Autodesk Inventor part; units mm, degrees
(part 2 of 2)
sketch "Skizze6" plane through (0, 0, -1.5) normal (0, 0, -1) x (-1, 0, 0)
  arc A0 (49.257, 13.1596) -> (46.9701, 10.7429) centre (49.9272, 10.235) ccw projected
  line L0 (49.257, 13.1596) -> (61.5242, 15.8801) projected
  arc A1 (63.0188, 15.8297) -> (61.5242, 15.8801) centre (62.1736, 12.9516) ccw projected
  line L1 (63.0188, 15.8297) -> (83.4642, 9.8255) projected
  arc A2 (83.4642, 9.8255) -> (85.086, 9.8061) centre (84.3096, 12.7044) ccw projected
  line L2 (85.086, 9.8061) -> (103.3977, 14.7128) projected
  arc A3 (103.3977, 14.7128) -> (105.5192, 18.3871) centre (102.6211, 17.6108) ccw projected
  line L3 (105.5192, 18.3871) -> (91.019, 72.5018) projected
  arc A4 (91.019, 72.5018) -> (88.8338, 74.6394) centre (88.1214, 71.7253) ccw projected
  line L4 (88.8338, 74.6394) -> (63.1786, 80.9125) projected
  arc A5 (63.1786, 80.9125) -> (62.6219, 80.9928) centre (62.4855, 78.0777) ccw projected
  line L5 (62.6219, 80.9928) -> (42.9227, 81.9679) projected
  arc A6 (42.9227, 81.9679) -> (41.7484, 81.7906) centre (42.7745, 78.9724) ccw projected
  line L6 (41.7484, 81.7906) -> (21.3272, 74.3579) projected
  arc A7 (21.3272, 74.3579) -> (20.5259, 73.9182) centre (22.3538, 71.5374) ccw projected
  line L7 (20.5259, 73.9182) -> (5.3305, 62.2476) projected
  arc A8 (4.8188, 61.9306) -> (5.3305, 62.2476) centre (3.5014, 64.629) ccw projected
  line L8 (4.8188, 61.9306) -> (-10.8605, 54.2803) projected
  arc A9 (-12.7723, 53.6855) -> (-10.8605, 54.2803) centre (-13.7536, 60.2096) ccw projected
  line L9 (-12.7723, 53.6855) -> (-36.149, 53.6855) projected
  arc A10 (-38.0608, 54.2803) -> (-36.149, 53.6855) centre (-36.149, 57.0556) ccw projected
  line L10 (-38.0608, 54.2803) -> (-53.7401, 61.9306) projected
  arc A11 (-54.2518, 62.2476) -> (-53.7401, 61.9306) centre (-52.4258, 64.6241) ccw projected
  line L11 (-54.2518, 62.2476) -> (-69.4472, 73.9182) projected
  arc A12 (-69.4472, 73.9182) -> (-70.2485, 74.3579) centre (-71.2736, 71.5402) ccw projected
  line L12 (-70.2485, 74.3579) -> (-90.6697, 81.7906) projected
  arc A13 (-90.6697, 81.7906) -> (-91.8441, 81.9679) centre (-91.696, 78.9707) ccw projected
  line L13 (-91.8441, 81.9679) -> (-111.5432, 80.9928) projected
  arc A14 (-111.5432, 80.9928) -> (-112.0999, 80.9125) centre (-111.3949, 77.9952) ccw projected
  line L14 (-112.0999, 80.9125) -> (-137.7551, 74.6394) projected
  arc A15 (-137.7551, 74.6394) -> (-139.9403, 72.5018) centre (-137.0425, 71.7251) ccw projected
  line L15 (-139.9403, 72.5018) -> (-154.4405, 18.3871) projected
  arc A16 (-154.4405, 18.3871) -> (-152.319, 14.7128) centre (-151.5428, 17.6106) ccw projected
  line L16 (-152.319, 14.7128) -> (-134.0073, 9.8061) projected
  arc A17 (-134.0073, 9.8061) -> (-132.3855, 9.8255) centre (-133.2309, 12.7035) ccw projected
  line L17 (-132.3855, 9.8255) -> (-111.9401, 15.8297) projected
  arc A18 (-110.4455, 15.8801) -> (-111.9401, 15.8297) centre (-111.0949, 12.9519) ccw projected
  line L18 (-110.4455, 15.8801) -> (-98.1783, 13.1596) projected
  arc A19 (-95.8914, 10.7429) -> (-98.1783, 13.1596) centre (-98.8211, 10.2609) ccw projected
  line L19 (-95.8914, 10.7429) -> (-92.4348, -9.3825) projected
  arc A20 (-92.4348, -9.3825) -> (-90.4875, -11.6997) centre (-89.4782, -8.8747) ccw projected
  line L20 (-90.4875, -11.6997) -> (-74.5563, -17.3936) projected
  arc A21 (-72.7201, -18.4315) -> (-74.5563, -17.3936) centre (-76.6396, -23.2223) ccw projected
  line L21 (-72.7201, -18.4315) -> (-58.4773, -34.2497) projected
  arc A22 (-57.7859, -35.5723) -> (-58.4773, -34.2497) centre (-60.7074, -36.2577) ccw projected
  line L22 (-57.7859, -35.5723) -> (-53.938, -51.3943) projected
  arc A23 (-53.938, -51.3943) -> (-50.2976, -53.5965) centre (-51.0229, -50.6854) ccw projected
  line L23 (-50.2976, -53.5965) -> (-31.4601, -48.8997) projected
  arc A24 (-30.7343, -48.8106) -> (-31.4601, -48.8997) centre (-30.7343, -51.8105) ccw projected
  line L24 (-30.7343, -48.8106) -> (-18.187, -48.8106) projected
  arc A25 (-17.4612, -48.8997) -> (-18.187, -48.8106) centre (-18.187, -51.8105) ccw projected
  line L25 (-17.4612, -48.8997) -> (1.3763, -53.5965) projected
  arc A26 (1.3763, -53.5965) -> (5.0167, -51.3943) centre (2.1019, -50.686) ccw projected
  line L26 (5.0167, -51.3943) -> (8.8645, -35.5723) projected
  arc A27 (9.556, -34.2497) -> (8.8645, -35.5723) centre (11.8759, -36.3046) ccw projected
  line L27 (9.556, -34.2497) -> (23.7988, -18.4315) projected
  arc A28 (25.635, -17.3936) -> (23.7988, -18.4315) centre (26.2659, -20.6529) ccw projected
  line L28 (25.635, -17.3936) -> (41.5662, -11.6997) projected
  arc A29 (41.5662, -11.6997) -> (43.5135, -9.3825) centre (40.5563, -8.8742) ccw projected
  line L29 (43.5135, -9.3825) -> (46.9701, 10.7429) projected
  line L30 (96.6013, 36.5996) -> (82.1125, 32.7172) projected
  line L31 (82.1125, 32.7172) -> (78.2301, 47.2061) projected
  line L32 (78.2301, 47.2061) -> (92.719, 51.0885) projected
  line L33 (92.719, 51.0885) -> (96.6013, 36.5996) projected
  line L34 (45.117, 62.9038) -> (31.0217, 57.7735) projected
  line L35 (31.0217, 57.7735) -> (25.8914, 71.8689) projected
  line L36 (25.8914, 71.8689) -> (39.9867, 76.9992) projected
  line L37 (39.9867, 76.9992) -> (45.117, 62.9038) projected
  line L38 (21.718, 27.7828) -> (16.5877, 41.8782) projected
  line L39 (16.5877, 41.8782) -> (30.6831, 47.0085) projected
  line L40 (30.6831, 47.0085) -> (35.8134, 32.9131) projected
  line L41 (35.8134, 32.9131) -> (21.718, 27.7828) projected
  line L42 (5.916, 15.6462) -> (20.0113, 20.7765) projected
  line L43 (20.0113, 20.7765) -> (25.1417, 6.6811) projected
  line L44 (25.1417, 6.6811) -> (11.0463, 1.5508) projected
  line L45 (11.0463, 1.5508) -> (5.916, 15.6462) projected
  line L46 (18.6433, 24.5353) -> (4.5479, 19.405) projected
  line L47 (4.5479, 19.405) -> (-0.5824, 33.5004) projected
  line L48 (-0.5824, 33.5004) -> (13.513, 38.6307) projected
  line L49 (13.513, 38.6307) -> (18.6433, 24.5353) projected
  line L50 (15.2196, 45.6369) -> (10.0893, 59.7323) projected
  line L51 (10.0893, 59.7323) -> (24.1847, 64.8626) projected
  line L52 (24.1847, 64.8626) -> (29.315, 50.7672) projected
  line L53 (29.315, 50.7672) -> (15.2196, 45.6369) projected
  line L54 (64.6087, 21.046) -> (59.4784, 35.1414) projected
  line L55 (59.4784, 35.1414) -> (73.5738, 40.2717) projected
  line L56 (73.5738, 40.2717) -> (78.7041, 26.1763) projected
  line L57 (78.7041, 26.1763) -> (64.6087, 21.046) projected
  line L58 (91.6837, 54.9522) -> (77.1948, 51.0698) projected
  line L59 (77.1948, 51.0698) -> (73.3125, 65.5587) projected
  line L60 (73.3125, 65.5587) -> (87.8013, 69.441) projected
  line L61 (87.8013, 69.441) -> (91.6837, 54.9522) projected
  line L62 (51.612, 56.7543) -> (46.4817, 70.8497) projected
  line L63 (46.4817, 70.8497) -> (60.5771, 75.98) projected
  line L64 (60.5771, 75.98) -> (65.7074, 61.8846) projected
  line L65 (65.7074, 61.8846) -> (51.612, 56.7543) projected
  line L66 (51.6154, 45.0496) -> (37.52, 39.9193) projected
  line L67 (37.52, 39.9193) -> (32.3897, 54.0147) projected
  line L68 (32.3897, 54.0147) -> (46.4851, 59.145) projected
  line L69 (46.4851, 59.145) -> (51.6154, 45.0496) projected
  line L70 (23.0861, 24.024) -> (37.1815, 29.1543) projected
  line L71 (37.1815, 29.1543) -> (42.3118, 15.0589) projected
  line L72 (42.3118, 15.0589) -> (28.2164, 9.9286) projected
  line L73 (28.2164, 9.9286) -> (23.0861, 24.024) projected
  line L74 (19.0184, 0.2419) -> (33.1433, 5.2903) projected
  line L75 (33.1433, 5.2903) -> (38.1917, -8.8346) projected
  line L76 (38.1917, -8.8346) -> (24.0668, -13.883) projected
  line L77 (24.0668, -13.883) -> (19.0184, 0.2419) projected
  line L78 (12.1449, 42.3895) -> (-1.9505, 37.2592) projected
  line L79 (-1.9505, 37.2592) -> (-7.0808, 51.3545) projected
  line L80 (-7.0808, 51.3545) -> (7.0146, 56.4848) projected
  line L81 (7.0146, 56.4848) -> (12.1449, 42.3895) projected
  line L82 (38.8881, 36.1605) -> (52.9835, 41.2908) projected
  line L83 (52.9835, 41.2908) -> (58.1138, 27.1954) projected
  line L84 (58.1138, 27.1954) -> (44.0184, 22.0651) projected
  line L85 (44.0184, 22.0651) -> (38.8881, 36.1605) projected
  line L86 (58.1104, 38.9001) -> (52.9801, 52.9955) projected
  line L87 (52.9801, 52.9955) -> (67.0754, 58.1258) projected
  line L88 (67.0754, 58.1258) -> (72.2057, 44.0304) projected
  line L89 (72.2057, 44.0304) -> (58.1104, 38.9001) projected
  line L90 (83.1478, 28.8535) -> (97.6366, 32.7359) projected
  line L91 (97.6366, 32.7359) -> (101.519, 18.247) projected
  line L92 (101.519, 18.247) -> (87.0301, 14.3647) projected
  line L93 (87.0301, 14.3647) -> (83.1478, 28.8535) projected
  line L94 (-127.1514, 47.2061) -> (-131.0338, 32.7172) projected
  line L95 (-131.0338, 32.7172) -> (-145.5226, 36.5996) projected
  line L96 (-145.5226, 36.5996) -> (-141.6403, 51.0885) projected
  line L97 (-141.6403, 51.0885) -> (-127.1514, 47.2061) projected
  line L98 (-74.8127, 71.8689) -> (-79.943, 57.7735) projected
  line L99 (-79.943, 57.7735) -> (-94.0383, 62.9038) projected
  line L100 (-94.0383, 62.9038) -> (-88.908, 76.9992) projected
  line L101 (-88.908, 76.9992) -> (-74.8127, 71.8689) projected
  line L102 (-79.6044, 47.0085) -> (-65.509, 41.8782) projected
  line L103 (-65.509, 41.8782) -> (-70.6393, 27.7828) projected
  line L104 (-70.6393, 27.7828) -> (-84.7347, 32.9131) projected
  line L105 (-84.7347, 32.9131) -> (-79.6044, 47.0085) projected
  line L106 (-74.063, 6.6811) -> (-68.9327, 20.7765) projected
  line L107 (-68.9327, 20.7765) -> (-54.8373, 15.6462) projected
  line L108 (-54.8373, 15.6462) -> (-59.9676, 1.5508) projected
  line L109 (-59.9676, 1.5508) -> (-74.063, 6.6811) projected
  line L110 (-48.3389, 33.5004) -> (-53.4692, 19.405) projected
  line L111 (-53.4692, 19.405) -> (-67.5646, 24.5353) projected
  line L112 (-67.5646, 24.5353) -> (-62.4343, 38.6307) projected
  line L113 (-62.4343, 38.6307) -> (-48.3389, 33.5004) projected
  line L114 (-73.106, 64.8626) -> (-59.0106, 59.7323) projected
  line L115 (-59.0106, 59.7323) -> (-64.1409, 45.6369) projected
  line L116 (-64.1409, 45.6369) -> (-78.2363, 50.7672) projected
  line L117 (-78.2363, 50.7672) -> (-73.106, 64.8626) projected
  line L118 (-122.4951, 40.2717) -> (-108.3997, 35.1414) projected
  line L119 (-108.3997, 35.1414) -> (-113.53, 21.046) projected
  line L120 (-113.53, 21.046) -> (-127.6254, 26.1763) projected
  line L121 (-127.6254, 26.1763) -> (-122.4951, 40.2717) projected
  line L122 (-122.2338, 65.5587) -> (-126.1161, 51.0698) projected
  line L123 (-126.1161, 51.0698) -> (-140.605, 54.9522) projected
  line L124 (-140.605, 54.9522) -> (-136.7226, 69.441) projected
  line L125 (-136.7226, 69.441) -> (-122.2338, 65.5587) projected
  line L126 (-109.4984, 75.98) -> (-95.403, 70.8497) projected
  line L127 (-95.403, 70.8497) -> (-100.5333, 56.7543) projected
  line L128 (-100.5333, 56.7543) -> (-114.6287, 61.8846) projected
  line L129 (-114.6287, 61.8846) -> (-109.4984, 75.98) projected
  line L130 (-81.311, 54.0147) -> (-86.4413, 39.9193) projected
  line L131 (-86.4413, 39.9193) -> (-100.5367, 45.0496) projected
  line L132 (-100.5367, 45.0496) -> (-95.4064, 59.145) projected
  line L133 (-95.4064, 59.145) -> (-81.311, 54.0147) projected
  line L134 (-91.2331, 15.0589) -> (-86.1028, 29.1543) projected
  line L135 (-86.1028, 29.1543) -> (-72.0074, 24.024) projected
  line L136 (-72.0074, 24.024) -> (-77.1377, 9.9286) projected
  line L137 (-77.1377, 9.9286) -> (-91.2331, 15.0589) projected
  line L138 (-87.113, -8.8346) -> (-82.0646, 5.2903) projected
  line L139 (-82.0646, 5.2903) -> (-67.9397, 0.2419) projected
  line L140 (-67.9397, 0.2419) -> (-72.9881, -13.883) projected
  line L141 (-72.9881, -13.883) -> (-87.113, -8.8346) projected
  line L142 (-41.8405, 51.3545) -> (-46.9708, 37.2592) projected
  line L143 (-46.9708, 37.2592) -> (-61.0662, 42.3895) projected
  line L144 (-61.0662, 42.3895) -> (-55.9359, 56.4848) projected
  line L145 (-55.9359, 56.4848) -> (-41.8405, 51.3545) projected
  line L146 (-107.0351, 27.1954) -> (-101.9048, 41.2908) projected
  line L147 (-101.9048, 41.2908) -> (-87.8094, 36.1605) projected
  line L148 (-87.8094, 36.1605) -> (-92.9397, 22.0651) projected
  line L149 (-92.9397, 22.0651) -> (-107.0351, 27.1954) projected
  line L150 (-115.9967, 58.1258) -> (-101.9014, 52.9955) projected
  line L151 (-101.9014, 52.9955) -> (-107.0317, 38.9001) projected
  line L152 (-107.0317, 38.9001) -> (-121.1271, 44.0304) projected
  line L153 (-121.1271, 44.0304) -> (-115.9967, 58.1258) projected
  line L154 (-150.4403, 18.247) -> (-146.5579, 32.7359) projected
  line L155 (-146.5579, 32.7359) -> (-132.0691, 28.8535) projected
  line L156 (-132.0691, 28.8535) -> (-135.9514, 14.3647) projected
  line L157 (-135.9514, 14.3647) -> (-150.4403, 18.247) projected
  circle A30 centre (-24.4607, 26.6625) radius 2.4143 projected
  line L158 (-13.01, 25.0985) -> (-22.3451, 15.7939) projected
  line L159 (-22.3451, 15.7939) -> (-24.1571, 17.6119) projected
  line L160 (-24.1571, 17.6119) -> (-14.822, 26.9165) projected
  line L161 (-14.822, 26.9165) -> (-13.01, 25.0985) projected
  line L162 (-14.6508, 7.2913) -> (-16.4993, 5.4489) projected
  line L163 (-16.4993, 5.4489) -> (-21.9532, 10.9208) projected
  line L164 (-21.9532, 10.9208) -> (-20.1048, 12.7631) projected
  line L165 (-20.1048, 12.7631) -> (-14.6508, 7.2913) projected
  line L166 (-12.4175, 9.5173) -> (-14.2593, 7.6816) projected
  line L167 (-14.2593, 7.6816) -> (-19.7132, 13.1534) projected
  line L168 (-19.7132, 13.1534) -> (-17.8714, 14.9892) projected
  line L169 (-17.8714, 14.9892) -> (-12.4175, 9.5173) projected
  line L170 (-15.2253, 27.342) -> (-22.2848, 20.2085) projected
  line L171 (-22.2848, 20.2085) -> (-24.1171, 22.0219) projected
  line L172 (-24.1171, 22.0219) -> (-17.0576, 29.1553) projected
  line L173 (-17.0576, 29.1553) -> (-15.2253, 27.342) projected
  line L174 (-10.7891, 22.8703) -> (-22.3642, 11.3331) projected
  line L175 (-22.3642, 11.3331) -> (-24.1705, 13.1453) projected
  line L176 (-24.1705, 13.1453) -> (-12.5954, 24.6825) projected
  line L177 (-12.5954, 24.6825) -> (-10.7891, 22.8703) projected
  line L178 (-16.8537, 5.1044) -> (-18.6469, 3.2872) projected
  line L179 (-18.6469, 3.2872) -> (-24.1171, 8.6849) projected
  line L180 (-24.1171, 8.6849) -> (-22.324, 10.5022) projected
  line L181 (-22.324, 10.5022) -> (-16.8537, 5.1044) projected
  line L182 (-8.5628, 20.6367) -> (-15.6177, 13.605) projected
  line L183 (-15.6177, 13.605) -> (-17.4329, 15.4262) projected
  line L184 (-17.4329, 15.4262) -> (-10.3781, 22.458) projected
  line L185 (-10.3781, 22.458) -> (-8.5628, 20.6367) projected
  line L186 (-26.5762, 15.7939) -> (-35.9113, 25.0985) projected
  line L187 (-35.9113, 25.0985) -> (-34.0993, 26.9165) projected
  line L188 (-34.0993, 26.9165) -> (-24.7642, 17.6119) projected
  line L189 (-24.7642, 17.6119) -> (-26.5762, 15.7939) projected
  line L190 (-32.422, 5.4489) -> (-34.2705, 7.2913) projected
  line L191 (-34.2705, 7.2913) -> (-28.8165, 12.7631) projected
  line L192 (-28.8165, 12.7631) -> (-26.9681, 10.9208) projected
  line L193 (-26.9681, 10.9208) -> (-32.422, 5.4489) projected
  line L194 (-34.662, 7.6816) -> (-36.5038, 9.5173) projected
  line L195 (-36.5038, 9.5173) -> (-31.0499, 14.9892) projected
  line L196 (-31.0499, 14.9892) -> (-29.2081, 13.1534) projected
  line L197 (-29.2081, 13.1534) -> (-34.662, 7.6816) projected
  line L198 (-26.6365, 20.2085) -> (-33.696, 27.342) projected
  line L199 (-33.696, 27.342) -> (-31.8637, 29.1553) projected
  line L200 (-31.8637, 29.1553) -> (-24.8042, 22.0219) projected
  line L201 (-24.8042, 22.0219) -> (-26.6365, 20.2085) projected
  line L202 (-26.5571, 11.3331) -> (-38.1322, 22.8703) projected
  line L203 (-38.1322, 22.8703) -> (-36.3259, 24.6825) projected
  line L204 (-36.3259, 24.6825) -> (-24.7508, 13.1453) projected
  line L205 (-24.7508, 13.1453) -> (-26.5571, 11.3331) projected
  line L206 (-30.2744, 3.2872) -> (-32.0676, 5.1044) projected
  line L207 (-32.0676, 5.1044) -> (-26.5973, 10.5022) projected
  line L208 (-26.5973, 10.5022) -> (-24.8042, 8.6849) projected
  line L209 (-24.8042, 8.6849) -> (-30.2744, 3.2872) projected
  line L210 (-33.3036, 13.605) -> (-40.3585, 20.6367) projected
  line L211 (-40.3585, 20.6367) -> (-38.5432, 22.458) projected
  line L212 (-38.5432, 22.458) -> (-31.4884, 15.4262) projected
  line L213 (-31.4884, 15.4262) -> (-33.3036, 13.605) projected
  line L214 (-54.0136, -35.0444) -> (-39.4592, -31.4155) projected
  line L215 (-39.4592, -31.4155) -> (-35.8303, -45.97) projected
  line L216 (-35.8303, -45.97) -> (-50.3848, -49.5988) projected
  line L217 (-50.3848, -49.5988) -> (-54.0136, -35.0444) projected
  line L218 (-67.7189, -18.1574) -> (-56.5717, -8.1205) projected
  line L219 (-56.5717, -8.1205) -> (-46.5348, -19.2676) projected
  line L220 (-46.5348, -19.2676) -> (-57.682, -29.3046) projected
  line L221 (-57.682, -29.3046) -> (-67.7189, -18.1574) projected
  line L222 (-9.4622, -31.4155) -> (5.0923, -35.0444) projected
  line L223 (5.0923, -35.0444) -> (1.4635, -49.5988) projected
  line L224 (1.4635, -49.5988) -> (-13.091, -45.97) projected
  line L225 (-13.091, -45.97) -> (-9.4622, -31.4155) projected
  line L226 (7.6504, -8.1205) -> (18.7976, -18.1574) projected
  line L227 (18.7976, -18.1574) -> (8.7607, -29.3046) projected
  line L228 (8.7607, -29.3046) -> (-2.3865, -19.2676) projected
  line L229 (-2.3865, -19.2676) -> (7.6504, -8.1205) projected
  point P0 (0, 0)
extrude "Extrusion4" add sketch "Skizze6" against normal blind 0.5 contours A30 | L158 L159 L160 L161 | L162 L163 L164 L165 | L166 L167 L168 L169 | L170 L171 L172 L173 | L174 L175 L176 L177 | L178 L179 L180 L181 | L182 L183 L184 L185 | L186 L187 L188 L189 | L190 L191 L192 L193 | L194 L195 L196 L197 | L198 L199 L200 L201 | L202 L203 L204 L205 | L206 L207 L208 L209 | L210 L211 L212 L213
sketch "Skizze7" plane through (0, 0, -1.5) normal (0, 0, -1) x (-1, 0, 0)
  circle A0 centre (-24.4607, -40.5072) radius 2.5 projected
  circle A1 centre (-24.4607, -40.5072) radius 1.1 projected
  circle A2 centre (-48.3814, 5.3151) radius 2.5 projected
  circle A3 centre (-48.3814, 5.3151) radius 1.1 projected
  circle A4 centre (-0.5399, 5.3151) radius 2.5 projected
  circle A5 centre (-0.5399, 5.3151) radius 1.45 projected
  arc A6 (-10.9742, 42.8975) -> (-10.3691, 41.235) centre (-11.7513, 41.6733) ccw projected
  arc A7 (-11.431, 44.1527) -> (-9.9122, 39.9798) centre (-11.7513, 41.6733) ccw projected
  arc A8 (-38.5522, 41.2349) -> (-37.9471, 42.8975) centre (-37.1701, 41.6733) ccw projected
  arc A9 (-39.0091, 39.9798) -> (-37.4903, 44.1527) centre (-37.1701, 41.6733) ccw projected
  circle A10 centre (-90.51, 4.4732) radius 1.45 projected
  circle A11 centre (-90.51, 4.4732) radius 2.5 projected
  circle A12 centre (-120.1445, 72.9705) radius 2.5 projected
  circle A13 centre (-127.5561, 15.9457) radius 2.5 projected
  circle A14 centre (-90.51, 4.4732) radius 2.5 projected
  line L0 (-145.5226, 36.5996) -> (-131.0338, 32.7172) projected
  line L1 (-141.6403, 51.0885) -> (-145.5226, 36.5996) projected
  line L2 (-127.1514, 47.2061) -> (-141.6403, 51.0885) projected
  line L3 (-131.0338, 32.7172) -> (-127.1514, 47.2061) projected
  line L4 (-94.0383, 62.9038) -> (-79.943, 57.7735) projected
  line L5 (-88.908, 76.9992) -> (-94.0383, 62.9038) projected
  line L6 (-74.8127, 71.8689) -> (-88.908, 76.9992) projected
  line L7 (-79.943, 57.7735) -> (-74.8127, 71.8689) projected
  line L8 (-70.6393, 27.7828) -> (-65.509, 41.8782) projected
  line L9 (-84.7347, 32.9131) -> (-70.6393, 27.7828) projected
  line L10 (-79.6044, 47.0085) -> (-84.7347, 32.9131) projected
  line L11 (-65.509, 41.8782) -> (-79.6044, 47.0085) projected
  line L12 (-54.8373, 15.6462) -> (-68.9327, 20.7765) projected
  line L13 (-59.9676, 1.5508) -> (-54.8373, 15.6462) projected
  line L14 (-74.063, 6.6811) -> (-59.9676, 1.5508) projected
  line L15 (-68.9327, 20.7765) -> (-74.063, 6.6811) projected
  line L16 (-67.5646, 24.5353) -> (-53.4692, 19.405) projected
  line L17 (-62.4343, 38.6307) -> (-67.5646, 24.5353) projected
  line L18 (-48.3389, 33.5004) -> (-62.4343, 38.6307) projected
  line L19 (-53.4692, 19.405) -> (-48.3389, 33.5004) projected
  line L20 (-64.1409, 45.6369) -> (-59.0106, 59.7323) projected
  line L21 (-78.2363, 50.7672) -> (-64.1409, 45.6369) projected
  line L22 (-73.106, 64.8626) -> (-78.2363, 50.7672) projected
  line L23 (-59.0106, 59.7323) -> (-73.106, 64.8626) projected
  line L24 (-113.53, 21.046) -> (-108.3997, 35.1414) projected
  line L25 (-127.6254, 26.1763) -> (-113.53, 21.046) projected
  line L26 (-122.4951, 40.2717) -> (-127.6254, 26.1763) projected
  line L27 (-108.3997, 35.1414) -> (-122.4951, 40.2717) projected
  line L28 (-140.605, 54.9522) -> (-126.1161, 51.0698) projected
  line L29 (-136.7226, 69.441) -> (-140.605, 54.9522) projected
  line L30 (-122.2338, 65.5587) -> (-136.7226, 69.441) projected
  line L31 (-126.1161, 51.0698) -> (-122.2338, 65.5587) projected
  line L32 (-100.5333, 56.7543) -> (-95.403, 70.8497) projected
  line L33 (-114.6287, 61.8846) -> (-100.5333, 56.7543) projected
  line L34 (-109.4984, 75.98) -> (-114.6287, 61.8846) projected
  line L35 (-95.403, 70.8497) -> (-109.4984, 75.98) projected
  line L36 (-100.5367, 45.0496) -> (-86.4413, 39.9193) projected
  line L37 (-95.4064, 59.145) -> (-100.5367, 45.0496) projected
  line L38 (-81.311, 54.0147) -> (-95.4064, 59.145) projected
  line L39 (-86.4413, 39.9193) -> (-81.311, 54.0147) projected
  line L40 (-72.0074, 24.024) -> (-86.1028, 29.1543) projected
  line L41 (-77.1377, 9.9286) -> (-72.0074, 24.024) projected
  line L42 (-91.2331, 15.0589) -> (-77.1377, 9.9286) projected
  line L43 (-86.1028, 29.1543) -> (-91.2331, 15.0589) projected
  line L44 (-67.9397, 0.2419) -> (-82.0646, 5.2903) projected
  line L45 (-72.9881, -13.883) -> (-67.9397, 0.2419) projected
  line L46 (-87.113, -8.8346) -> (-72.9881, -13.883) projected
  line L47 (-82.0646, 5.2903) -> (-87.113, -8.8346) projected
  line L48 (-61.0662, 42.3895) -> (-46.9708, 37.2592) projected
  line L49 (-55.9359, 56.4848) -> (-61.0662, 42.3895) projected
  line L50 (-41.8405, 51.3545) -> (-55.9359, 56.4848) projected
  line L51 (-46.9708, 37.2592) -> (-41.8405, 51.3545) projected
  line L52 (-87.8094, 36.1605) -> (-101.9048, 41.2908) projected
  line L53 (-92.9397, 22.0651) -> (-87.8094, 36.1605) projected
  line L54 (-107.0351, 27.1954) -> (-92.9397, 22.0651) projected
  line L55 (-101.9048, 41.2908) -> (-107.0351, 27.1954) projected
  line L56 (-107.0317, 38.9001) -> (-101.9014, 52.9955) projected
  line L57 (-121.1271, 44.0304) -> (-107.0317, 38.9001) projected
  line L58 (-115.9967, 58.1258) -> (-121.1271, 44.0304) projected
  line L59 (-101.9014, 52.9955) -> (-115.9967, 58.1258) projected
  line L60 (-132.0691, 28.8535) -> (-146.5579, 32.7359) projected
  line L61 (-135.9514, 14.3647) -> (-132.0691, 28.8535) projected
  line L62 (-150.4403, 18.247) -> (-135.9514, 14.3647) projected
  line L63 (-146.5579, 32.7359) -> (-150.4403, 18.247) projected
  arc A15 (-69.4472, 73.9182) -> (-70.2485, 74.3579) centre (-71.2739, 71.5396) ccw projected
  line L64 (-90.6697, 81.7906) -> (-70.2485, 74.3579) projected
  arc A16 (-90.6697, 81.7906) -> (-91.8441, 81.9679) centre (-91.6959, 78.9716) ccw projected
  line L65 (-111.5432, 80.9928) -> (-91.8441, 81.9679) projected
  arc A17 (-111.5432, 80.9928) -> (-112.0999, 80.9125) centre (-111.3949, 77.9956) ccw projected
  line L66 (-137.7551, 74.6394) -> (-112.0999, 80.9125) projected
  arc A18 (-137.7551, 74.6394) -> (-139.9403, 72.5018) centre (-137.0429, 71.7256) ccw projected
  line L67 (-154.4405, 18.3871) -> (-139.9403, 72.5018) projected
  arc A19 (-154.4405, 18.3871) -> (-152.319, 14.7128) centre (-151.5429, 17.6106) ccw projected
  line L68 (-134.0073, 9.8061) -> (-152.319, 14.7128) projected
  arc A20 (-134.0073, 9.8061) -> (-132.3855, 9.8255) centre (-133.2309, 12.7036) ccw projected
  line L69 (-111.9401, 15.8297) -> (-132.3855, 9.8255) projected
  arc A21 (-110.4455, 15.8801) -> (-111.9401, 15.8297) centre (-111.0949, 12.9516) ccw projected
  line L70 (-98.1783, 13.1596) -> (-110.4455, 15.8801) projected
  arc A22 (-95.8914, 10.7429) -> (-98.1783, 13.1596) centre (-98.8479, 10.2356) ccw projected
  line L71 (-92.4348, -9.3825) -> (-95.8914, 10.7429) projected
  arc A23 (-92.4348, -9.3825) -> (-90.4875, -11.6997) centre (-89.4779, -8.8744) ccw projected
  line L72 (-74.5563, -17.3936) -> (-90.4875, -11.6997) projected
  line L73 (-59.0742, -3.4534) -> (-74.5563, -17.3936) projected
  line L74 (-38.0608, 54.2803) -> (-59.0742, -3.4534) projected
  line L75 (-53.7401, 61.9306) -> (-38.0608, 54.2803) projected
  arc A24 (-54.2518, 62.2476) -> (-53.7401, 61.9306) centre (-52.4249, 64.6256) ccw projected
  line L76 (-69.4472, 73.9182) -> (-54.2518, 62.2476) projected
  circle A25 centre (-127.5561, 15.9457) radius 1.45 projected
  circle A26 centre (-120.1445, 72.9705) radius 1.45 projected
  circle A27 centre (71.2232, 72.9705) radius 1.45 projected
  circle A28 centre (71.2232, 72.9705) radius 1.45 projected
  circle A29 centre (71.2232, 72.9705) radius 2.5 projected
  circle A30 centre (78.6348, 15.9457) radius 2.5 projected
  circle A31 centre (78.6348, 15.9457) radius 1.45 projected
  circle A32 centre (41.5887, 4.4732) radius 2.5 projected
  circle A33 centre (41.5887, 4.4732) radius 2.5 projected
  circle A34 centre (41.5887, 4.4732) radius 1.45 projected
  circle A35 centre (-11.7513, 41.6733) radius 1.45
  circle A36 centre (-11.7513, 41.6733) radius 2.5
  circle A37 centre (-37.1701, 41.6733) radius 1.45
  circle A38 centre (-37.1701, 41.6733) radius 2.5
  circle A39 centre (-48.3814, 5.3151) radius 1.45
  circle A40 centre (-24.4607, -40.5072) radius 1.45
  point P0 (0, 0)
  point P1 (-39.0091, 39.9798)
  point P2 (-38.5522, 41.2349)
  point P3 (-37.9471, 42.8975)
  point P4 (-9.9122, 39.9798)
  point P5 (-10.3691, 41.235)
  point P6 (-10.9742, 42.8975)
  dimension "d13" = 2.9
  dimension "d14" = 2.9
  constraints: 6 centre point, 6 coincident, 4 concentric
  measures "d13" diameter of A39
  measures "d14" diameter of A40
extrude "Extrusion5" add sketch "Skizze7" along normal blind 3.5 contours A0 | A2 | A4 | A36 A7 | A38 A9 | A11 | A12 | A13 | A29 | A30 | A32
sketch "Skizze9" plane through (33.2927, 55.6855, -6.6) normal (0, 0, -1) x (-1, 0, 0)
  arc A0 (-104.4624, 18.9539) -> (-106.6476, 16.8163) centre (-103.7498, 16.0396) ccw projected
  line L0 (-78.8073, 25.227) -> (-104.4624, 18.9539) projected
  arc A1 (-78.2506, 25.3074) -> (-78.8073, 25.227) centre (-78.1022, 22.3098) ccw projected
  line L1 (-58.5514, 26.2824) -> (-78.2506, 25.3074) projected
  arc A2 (-57.377, 26.1051) -> (-58.5514, 26.2824) centre (-58.4034, 23.2853) ccw projected
  line L2 (-36.9558, 18.6725) -> (-57.377, 26.1051) projected
  arc A3 (-36.1545, 18.2327) -> (-36.9558, 18.6725) centre (-37.9809, 15.8547) ccw projected
  line L3 (-20.9592, 6.5621) -> (-36.1545, 18.2327) projected
  arc A4 (-20.9592, 6.5621) -> (-20.4474, 6.2451) centre (-19.1331, 8.9386) ccw projected
  line L4 (-4.7682, -1.4052) -> (-20.4474, 6.2451) projected
  arc A5 (-4.7682, -1.4052) -> (-2.8563, -2) centre (-2.8563, 1.3701) ccw projected
  line L5 (20.5203, -2) -> (-2.8563, -2) projected
  arc A6 (20.5203, -2) -> (22.4322, -1.4052) centre (19.5391, 4.5242) ccw projected
  line L6 (38.1114, 6.2451) -> (22.4322, -1.4052) projected
  arc A7 (38.1114, 6.2451) -> (38.6232, 6.5621) centre (36.7941, 8.9436) ccw projected
  line L7 (53.8186, 18.2327) -> (38.6232, 6.5621) projected
  arc A8 (54.6199, 18.6725) -> (53.8186, 18.2327) centre (55.6465, 15.8519) ccw projected
  line L8 (75.0411, 26.1051) -> (54.6199, 18.6725) projected
  arc A9 (76.2154, 26.2824) -> (75.0411, 26.1051) centre (76.0671, 23.2869) ccw projected
  line L9 (95.9146, 25.3074) -> (76.2154, 26.2824) projected
  arc A10 (96.4713, 25.227) -> (95.9146, 25.3074) centre (95.7781, 22.3922) ccw projected
  line L10 (122.1264, 18.9539) -> (96.4713, 25.227) projected
  arc A11 (124.3117, 16.8163) -> (122.1264, 18.9539) centre (121.4141, 16.0399) ccw projected
  line L11 (138.8119, -37.2984) -> (124.3117, 16.8163) projected
  arc A12 (136.6903, -40.9727) -> (138.8119, -37.2984) centre (135.9138, -38.0747) ccw projected
  line L12 (118.3786, -45.8793) -> (136.6903, -40.9727) projected
  arc A13 (116.7568, -45.8599) -> (118.3786, -45.8793) centre (117.6023, -42.9811) ccw projected
  line L13 (96.3114, -39.8557) -> (116.7568, -45.8599) projected
  arc A14 (96.3114, -39.8557) -> (94.8168, -39.8054) centre (95.4663, -42.7339) ccw projected
  line L14 (82.5496, -42.5259) -> (94.8168, -39.8054) projected
  arc A15 (82.5496, -42.5259) -> (80.2628, -44.9426) centre (83.2199, -45.4505) ccw projected
  line L15 (76.8061, -65.068) -> (80.2628, -44.9426) projected
  arc A16 (74.8588, -67.3851) -> (76.8061, -65.068) centre (73.849, -64.5597) ccw projected
  line L16 (58.9277, -73.0791) -> (74.8588, -67.3851) projected
  arc A17 (58.9277, -73.0791) -> (57.0915, -74.117) centre (59.5586, -76.3384) ccw projected
  line L17 (42.8487, -89.9352) -> (57.0915, -74.117) projected
  arc A18 (42.8487, -89.9352) -> (42.1572, -91.2578) centre (45.1685, -91.9901) ccw projected
  line L18 (38.3093, -107.0798) -> (42.1572, -91.2578) projected
  arc A19 (34.6689, -109.2819) -> (38.3093, -107.0798) centre (35.3946, -106.3715) ccw projected
  line L19 (15.8315, -104.5852) -> (34.6689, -109.2819) projected
  arc A20 (15.8315, -104.5852) -> (15.1057, -104.4961) centre (15.1057, -107.496) ccw projected
  line L20 (2.5583, -104.4961) -> (15.1057, -104.4961) projected
  arc A21 (2.5583, -104.4961) -> (1.8326, -104.5852) centre (2.5583, -107.496) ccw projected
  line L21 (-17.0049, -109.2819) -> (1.8326, -104.5852) projected
  arc A22 (-20.6453, -107.0798) -> (-17.0049, -109.2819) centre (-17.7302, -106.3709) ccw projected
  line L22 (-24.4932, -91.2578) -> (-20.6453, -107.0798) projected
  arc A23 (-24.4932, -91.2578) -> (-25.1846, -89.9352) centre (-27.4147, -91.9432) ccw projected
  line L23 (-39.4274, -74.117) -> (-25.1846, -89.9352) projected
  arc A24 (-39.4274, -74.117) -> (-41.2637, -73.0791) centre (-43.3469, -78.9078) ccw projected
  line L24 (-57.1948, -67.3851) -> (-41.2637, -73.0791) projected
  arc A25 (-59.1421, -65.068) -> (-57.1948, -67.3851) centre (-56.1855, -64.5602) ccw projected
  line L25 (-62.5987, -44.9426) -> (-59.1421, -65.068) projected
  arc A26 (-62.5987, -44.9426) -> (-64.8856, -42.5259) centre (-65.5284, -45.4245) ccw projected
  line L26 (-77.1528, -39.8054) -> (-64.8856, -42.5259) projected
  arc A27 (-77.1528, -39.8054) -> (-78.6474, -39.8557) centre (-77.8023, -42.7336) ccw projected
  line L27 (-99.0928, -45.8599) -> (-78.6474, -39.8557) projected
  arc A28 (-100.7146, -45.8793) -> (-99.0928, -45.8599) centre (-99.9382, -42.982) ccw projected
  line L28 (-119.0263, -40.9727) -> (-100.7146, -45.8793) projected
  arc A29 (-121.1479, -37.2984) -> (-119.0263, -40.9727) centre (-118.2501, -38.0748) ccw projected
  line L29 (-106.6476, 16.8163) -> (-121.1479, -37.2984) projected
  line L30 (-19.5602, 8.0376) -> (-3.8058, 0.3506) projected
  line L31 (-34.9362, 19.8188) -> (-19.5602, 8.0376) projected
  arc A30 (-34.9362, 19.8188) -> (-36.2715, 20.5517) centre (-37.9812, 15.8541) ccw projected
  line L32 (-56.6932, 27.9845) -> (-36.2715, 20.5517) projected
  arc A31 (-56.6932, 27.9845) -> (-58.6504, 28.28) centre (-58.4032, 23.2861) ccw projected
  line L33 (-78.2506, 27.3098) -> (-58.6504, 28.28) projected
  arc A32 (-78.2506, 27.3098) -> (-79.3001, 27.1654) centre (-77.95, 21.2374) ccw projected
  line L34 (-104.9377, 20.8966) -> (-79.3001, 27.1654) projected
  arc A33 (-104.9377, 20.8966) -> (-108.5794, 17.3341) centre (-103.7502, 16.0401) ccw projected
  line L35 (-123.0797, -36.7808) -> (-108.5794, 17.3341) projected
  arc A34 (-123.0797, -36.7808) -> (-119.5443, -42.9044) centre (-118.2502, -38.0749) ccw projected
  line L36 (-101.2323, -47.8112) -> (-119.5443, -42.9044) projected
  arc A35 (-101.2323, -47.8112) -> (-98.6442, -47.8112) centre (-99.9382, -42.9819) ccw projected
  line L37 (-78.0954, -41.7781) -> (-98.6442, -47.8112) projected
  arc A36 (-77.5858, -41.7579) -> (-78.0954, -41.7781) centre (-77.8003, -42.7832) ccw projected
  line L38 (-65.3388, -44.4739) -> (-77.5858, -41.7579) projected
  arc A37 (-64.5699, -45.2807) -> (-65.3388, -44.4739) centre (-65.5552, -45.4499) ccw projected
  line L39 (-61.1133, -65.4063) -> (-64.5699, -45.2807) projected
  arc A38 (-61.1133, -65.4063) -> (-57.8681, -69.2684) centre (-56.1852, -64.5599) ccw projected
  line L40 (-42.5675, -74.737) -> (-57.8681, -69.2684) projected
  arc A39 (-39.5756, -76.9413) -> (-42.5675, -74.737) centre (-44.7418, -80.8205) ccw projected
  line L41 (-26.6708, -91.2736) -> (-39.5756, -76.9413) projected
  arc A40 (-26.439, -91.7203) -> (-26.6708, -91.2736) centre (-27.4142, -91.9429) ccw projected
  line L42 (-22.5887, -107.5525) -> (-26.439, -91.7203) projected
  arc A41 (-22.5887, -107.5525) -> (-16.5206, -111.2224) centre (-17.7302, -106.3709) ccw projected
  line L43 (2.3169, -106.5257) -> (-16.5206, -111.2224) projected
  arc A42 (2.5733, -106.4961) -> (2.3169, -106.5257) centre (2.5588, -107.4959) ccw projected
  line L44 (15.0907, -106.4961) -> (2.5733, -106.4961) projected
  arc A43 (15.3472, -106.5257) -> (15.0907, -106.4961) centre (15.0907, -107.6222) ccw projected
  line L45 (34.1847, -111.2224) -> (15.3472, -106.5257) projected
  arc A44 (34.1847, -111.2224) -> (40.2527, -107.5525) centre (35.3943, -106.3709) ccw projected
  line L46 (44.103, -91.7203) -> (40.2527, -107.5525) projected
  arc A45 (44.3349, -91.2736) -> (44.103, -91.7203) centre (45.1311, -91.9703) ccw projected
  line L47 (57.2117, -76.9725) -> (44.3349, -91.2736) projected
  arc A46 (60.2315, -74.737) -> (57.2117, -76.9725) centre (64.2209, -83.2836) ccw projected
  line L48 (75.5321, -69.2684) -> (60.2315, -74.737) projected
  arc A47 (75.5321, -69.2684) -> (78.7773, -65.4063) centre (73.8493, -64.5599) ccw projected
  line L49 (82.234, -45.2807) -> (78.7773, -65.4063) projected
  arc A48 (83.0028, -44.4739) -> (82.234, -45.2807) centre (83.2193, -45.4499) ccw projected
  line L50 (95.2498, -41.7579) -> (83.0028, -44.4739) projected
  arc A49 (95.7594, -41.7781) -> (95.2498, -41.7579) centre (95.4663, -42.7339) ccw projected
  line L51 (116.1935, -47.779) -> (95.7594, -41.7781) projected
  arc A50 (116.1935, -47.779) -> (118.8963, -47.8112) centre (117.6023, -42.9819) ccw projected
  line L52 (137.2084, -42.9044) -> (118.8963, -47.8112) projected
  arc A51 (137.2084, -42.9044) -> (140.7438, -36.7808) centre (135.9143, -38.0749) ccw projected
  line L53 (126.2435, 17.3341) -> (140.7438, -36.7808) projected
  arc A52 (126.2435, 17.3341) -> (122.6018, 20.8966) centre (121.4128, 16.0385) ccw projected
  line L54 (96.9641, 27.1654) -> (122.6018, 20.8966) projected
  arc A53 (96.9641, 27.1654) -> (96.0135, 27.3049) centre (95.7503, 22.2015) ccw projected
  line L55 (76.3145, 28.28) -> (96.0135, 27.3049) projected
  arc A54 (76.3145, 28.28) -> (74.3572, 27.9845) centre (76.0673, 23.286) ccw projected
  line L56 (53.9364, 20.5522) -> (74.3572, 27.9845) projected
  arc A55 (53.9364, 20.5522) -> (52.6002, 19.8188) centre (55.6473, 15.8514) ccw projected
  line L57 (37.4047, 8.1479) -> (52.6002, 19.8188) projected
  line L58 (37.0846, 7.9695) -> (37.4047, 8.1479) projected
  line L59 (21.4698, 0.3506) -> (37.0846, 7.9695) projected
  arc A56 (17.664, 0) -> (21.4698, 0.3506) centre (17.664, 20.8319) ccw projected
  line L60 (0, 0) -> (17.664, 0) projected
  arc A57 (-3.8058, 0.3506) -> (0, 0) centre (0, 20.8319) ccw projected
  arc A58 (-104.6999, 19.9253) -> (-107.6136, 17.0749) centre (-103.7498, 16.0396) ccw
  line L61 (-107.6136, 17.0749) -> (-122.1138, -37.0395)
  arc A59 (-122.1138, -37.0395) -> (-119.2854, -41.9385) centre (-118.2501, -38.0748) ccw
  line L62 (-119.2854, -41.9385) -> (-100.9734, -46.8453)
  arc A60 (-100.9734, -46.8453) -> (-98.8113, -46.8195) centre (-99.9382, -42.982) ccw
  line L63 (-98.8113, -46.8195) -> (-78.3656, -40.8152)
  arc A61 (-77.3694, -40.7816) -> (-78.3656, -40.8152) centre (-77.8023, -42.7336) ccw
  line L64 (-77.3694, -40.7816) -> (-65.1021, -43.5022)
  arc A62 (-63.5849, -45.108) -> (-65.1021, -43.5022) centre (-65.5284, -45.4245) ccw
  line L65 (-63.5849, -45.108) -> (-60.1277, -65.2372)
  arc A63 (-60.1277, -65.2372) -> (-57.5317, -68.3267) centre (-56.1855, -64.5602) ccw
  line L66 (-57.5317, -68.3267) -> (-41.6002, -74.0207)
  arc A64 (-40.1173, -74.8452) -> (-41.6002, -74.0207) centre (-43.3469, -78.9078) ccw
  line L67 (-40.1173, -74.8452) -> (-25.9278, -90.6043)
  arc A65 (-25.4659, -91.4897) -> (-25.9278, -90.6043) centre (-27.4147, -91.9432) ccw
  line L68 (-25.4659, -91.4897) -> (-21.617, -107.3161)
  arc A66 (-21.617, -107.3161) -> (-16.7625, -110.2521) centre (-17.7302, -106.3709) ccw
  line L69 (-16.7625, -110.2521) -> (2.0745, -105.5555)
  arc A67 (2.5583, -105.4961) -> (2.0745, -105.5555) centre (2.5583, -107.496) ccw
  line L70 (2.5583, -105.4961) -> (15.1057, -105.4961)
  arc A68 (15.5895, -105.5555) -> (15.1057, -105.4961) centre (15.1057, -107.496) ccw
  line L71 (15.5895, -105.5555) -> (34.427, -110.2522)
  arc A69 (34.427, -110.2522) -> (39.2809, -107.3166) centre (35.3946, -106.3715) ccw
  line L72 (39.2809, -107.3166) -> (43.1289, -91.4941)
  arc A70 (43.5948, -90.601) -> (43.1289, -91.4941) centre (45.1685, -91.9901) ccw
  line L73 (43.5948, -90.601) -> (57.8346, -74.7861)
  arc A71 (59.1861, -74.0487) -> (57.8346, -74.7861) centre (59.5586, -76.3384) ccw
  line L74 (59.1861, -74.0487) -> (75.1954, -68.3268)
  arc A72 (75.1954, -68.3268) -> (77.7918, -65.2369) centre (73.849, -64.5597) ccw
  line L75 (77.7918, -65.2369) -> (81.2483, -45.1118)
  arc A73 (82.7699, -43.5013) -> (81.2483, -45.1118) centre (83.2199, -45.4505) ccw
  line L76 (82.7699, -43.5013) -> (95.0333, -40.7817)
  arc A74 (96.0297, -40.8153) -> (95.0333, -40.7817) centre (95.4663, -42.7339) ccw
  line L77 (96.0297, -40.8153) -> (116.4751, -46.8194)
  arc A75 (116.4751, -46.8194) -> (118.6377, -46.8452) centre (117.6023, -42.9811) ccw
  line L78 (118.6377, -46.8452) -> (136.9492, -41.9386)
  arc A76 (136.9492, -41.9386) -> (139.7778, -37.0393) centre (135.9138, -38.0747) ccw
  line L79 (139.7778, -37.0393) -> (125.2776, 17.0751)
  arc A77 (125.2776, 17.0751) -> (122.3641, 19.9252) centre (121.4141, 16.0399) ccw
  line L80 (122.3641, 19.9252) -> (96.7088, 26.1984)
  arc A78 (96.7088, 26.1984) -> (95.9628, 26.3062) centre (95.7781, 22.3922) ccw
  line L81 (95.9628, 26.3062) -> (76.2649, 27.2812)
  arc A79 (76.2649, 27.2812) -> (74.6994, 27.0449) centre (76.0671, 23.2869) ccw
  line L82 (74.6994, 27.0449) -> (54.2779, 19.6122)
  arc A80 (54.2779, 19.6122) -> (53.209, 19.0255) centre (55.6465, 15.8519) ccw
  line L83 (53.209, 19.0255) -> (38.0141, 7.3552)
  arc A81 (37.6724, 7.1436) -> (38.0141, 7.3552) centre (36.7941, 8.9436) ccw
  line L84 (37.6724, 7.1436) -> (21.9937, -0.5065)
  arc A82 (20.4425, -1) -> (21.9937, -0.5065) centre (19.5391, 4.5242) ccw
  line L85 (20.4425, -1) -> (-2.8563, -1)
  arc A83 (-4.2565, -0.5422) -> (-2.8563, -1) centre (-2.8563, 1.3701) ccw
  line L86 (-4.2565, -0.5422) -> (-20.0089, 7.1438)
  arc A84 (-20.3496, 7.3548) -> (-20.0089, 7.1438) centre (-19.1331, 8.9386) ccw
  line L87 (-20.3496, 7.3548) -> (-35.5454, 19.0258)
  arc A85 (-35.5454, 19.0258) -> (-36.6134, 19.612) centre (-37.9809, 15.8547) ccw
  line L88 (-36.6134, 19.612) -> (-57.035, 27.0448)
  arc A86 (-57.035, 27.0448) -> (-58.6012, 27.2812) centre (-58.4034, 23.2853) ccw
  line L89 (-58.6012, 27.2812) -> (-78.3, 26.3061)
  arc A87 (-78.3, 26.3061) -> (-79.0436, 26.1987) centre (-78.1022, 22.3098) ccw
  line L90 (-79.0436, 26.1987) -> (-104.6999, 19.9253)
  point P0 (33.2927, -55.6855)
  dimension "d10" = 1
  constraints: 60 end point, 60 point on circle, 30 centre point, 59 other
  measures "d10" distance between parallel lines of L0 L90
extrude "Extrusion6" cut sketch "Skizze9" against normal up to surface (1.6 mm away) contours L90 A87 L89 A86 L88 A85 L87 A84 L86 A83 L85 A82 L84 A81 L83 A80 L82 A79 L81 A78 L80 A77 L79 A76 L78 A75 L77 A74 L76 A73 L75 A72 L74 A71 L73 A70 L72 A69 L71 A68 L70 A67 L69 A66 L68 A65 L67 A64 L66 A63 L65 A62 L64 A61 L63 A60 L62 A59 L61 A58
